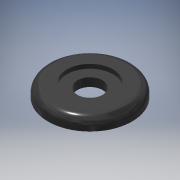
# Autodesk Inventor part: Component 15 (Hold Down Valve Spring)
Saved by Autodesk Inventor 2018 (Build 220112000, 112)
## iProperties
Created: 2023-03-14
Part Number: Component 15 (Hold Down Valve Spring)
Material: Generic
Document SubType Name: Modeling
Designer: Habib Mohamed
Density: 1 g/cm^3
Appearance: Dark Gray
Author: Habib Mohamed
Autodesk Inventor part; units mm, degrees
ref_plane "YZ Plane" through (0, 0, 0) normal (1, 0, 0) x (0, 1, 0)
ref_plane "XZ Plane" through (0, 0, 0) normal (0, 1, 0) x (-1, 0, 0)
ref_plane "XY Plane" through (0, 0, 0) normal (0, 0, 1) x (1, 0, 0)
sketch "Sketch1" plane through (0, 0, 0) normal (1, 0, 0) x (0, 1, 0)
  line L0 (0, 0) -> (4.0764, 0) construction
  line L1 (0, -1.5) -> (1, -1.5)
  line L2 (1, -1.5) -> (1, -2.75)
  line L3 (1, -2.75) -> (1.5, -2.75)
  line L4 (1.5, -2.75) -> (1.5, -4)
  line L5 (0.5, -5) -> (0, -5)
  line L6 (0, -5) -> (0, -4.5)
  line L7 (0, -4.5) -> (0.45, -4.5)
  line L8 (0.5, -4.45) -> (0.5, -3.55)
  line L9 (0.45, -3.5) -> (0, -3.5)
  line L10 (0, -3.5) -> (0, -1.5)
  arc A0 (0.5, -5) -> (1.5, -4) centre (0.5, -4) ccw
  arc A1 (0.5, -3.55) -> (0.45, -3.5) centre (0.45, -3.55) ccw
  arc A2 (0.45, -4.5) -> (0.5, -4.45) centre (0.45, -4.45) ccw
  point P0 (0.5, -4.5)
  dimension "d0" = 5
  dimension "d1" = 4.5
  dimension "d2" = 3.5
  dimension "d3" = 1.5
  dimension "d4" = 1.5
  dimension "d5" = 0.5
  dimension "d6" = 0.5
  dimension "d7" = 2.75
  dimension "d8" = 1
  dimension "d9" = 0.05
  constraints: 22 end point, 8 perpendicular, 6 point on circle, 6 tangent, 4 point on line, 3 centre point, 3 horizontal, 1 equal radius
  measures "d0" distance between parallel lines of L5 L0
  measures "d1" distance between parallel lines of L0 L7
  measures "d2" distance between parallel lines of L0 L9
  measures "d3" distance between parallel lines of L0 L1
  measures "d4" distance between parallel lines of L4 L6
  measures "d5" distance between parallel lines of L4 L2
  measures "d6" distance of L6.end point (0.5, -4.5)
  measures "d7" distance between parallel lines of L0 L3
  measures "d8" radius of A0
  measures "d9" radius of A1
revolve "Revolution1" add sketch "Sketch1" angle 360 about axis through (0, 0, 0) along (0, 1, 0)
body "Solid1"
